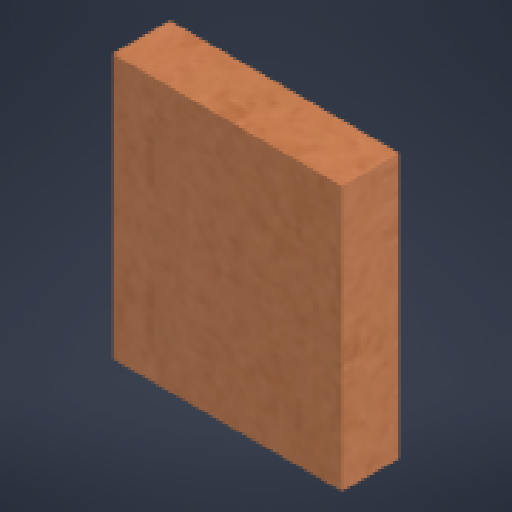
# Autodesk Inventor part: Servo Stand
Saved by Autodesk Inventor 2026.2 (Build 302298000, 298)
## iProperties
Created: 2026-04-11
Part Number: Servo Stand
Material: Wood (Walnut)
Document SubType Name: Modeling
Designer: abdul
Density: 0.55 g/cm^3
Appearance: Walnut - Natural Polished
Author: abdul
Autodesk Inventor part; units mm, degrees
ref_plane "YZ Plane" through (0, 0, 0) normal (1, 0, 0) x (0, 1, 0)
ref_plane "XZ Plane" through (0, 0, 0) normal (0, 1, 0) x (-1, 0, 0)
ref_plane "XY Plane" through (0, 0, 0) normal (0, 0, 1) x (1, 0, 0)
sketch "Sketch1" plane through (0, 0, 0) normal (0, 0, 1) x (1, 0, 0)
  line L0 (20, -23) -> (-20, -23)
  line L1 (-20, -23) -> (-20, 23)
  line L2 (-20, 23) -> (20, 23)
  line L3 (20, 23) -> (20, -23)
  line L4 (20, -23) -> (-20, 23) construction
  line L5 (-20, -23) -> (20, 23) construction
  line L6 (-10, -13) -> (10, -13)
  line L7 (10, -13) -> (10, 13)
  line L8 (10, 13) -> (-10, 13)
  line L9 (-10, 13) -> (-10, -13)
  point P0 (0, 0)
  dimension "d0" = 46
  dimension "d1" = 40
  dimension "d2" = 26
  constraints: 20 end point, 4 parallel, 2 midpoint, 2 perpendicular, 1 horizontal, 3 other
  measures "d0" distance of L2.end L0.start
  measures "d1" distance of L1.end L2.end
  measures "d2" distance of L6.end L7.end
extrude "Extrusion1" add sketch "Sketch1" along normal blind 5
extrude "Extrusion2" add sketch "Sketch1" along normal blind 5 contours L9 L8 L7 L6
body "Solid1"
